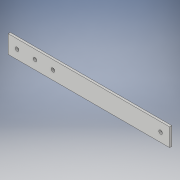
# Autodesk Inventor part: Gearbox Mounting Gusset
Saved by Autodesk Inventor 2018 (Build 220112000, 112)
## iProperties
Created: 2019-01-23
Part Number: Gearbox Mounting Gusset
Material: Generic
Document SubType Name: Modeling
Designer: Gabriel
Density: 1 g/cm^3
Appearance: Default
Author: Gabriel
Autodesk Inventor part; units mm, degrees
ref_plane "YZ Plane" through (0, 0, 0) normal (1, 0, 0) x (0, 1, 0)
ref_plane "XZ Plane" through (0, 0, 0) normal (0, 1, 0) x (-1, 0, 0)
ref_plane "XY Plane" through (0, 0, 0) normal (0, 0, 1) x (1, 0, 0)
sketch "Sketch1" plane through (0, 0, 0) normal (0, 0, 1) x (1, 0, 0)
  line L0 (-12.3524, -19.5597) -> (216.2476, -19.5597)
  line L1 (216.2476, -19.5597) -> (216.2476, -44.9597)
  line L2 (216.2476, -44.9597) -> (-12.3524, -44.9597)
  line L3 (-12.3524, -44.9597) -> (-12.3524, -19.5597)
  point P0 (0, 0)
  dimension "d0" = 228.6
  dimension "d1" = 25.4
  constraints: 8 end point, 2 parallel, 1 horizontal, 1 perpendicular
  measures "d0" distance of L1.end L2.end
  measures "d1" distance of L0.end L1.end
extrude "Extrusion1" add sketch "Sketch1" along normal blind 3.175
sketch "Sketch2" plane through (0, 0, 3.175) normal (0, 0, 1) x (1, 0, 0)
  line L0 (216.2476, -44.9597) -> (216.2476, -19.5597) construction
  line L1 (216.2476, -32.2597) -> (203.5476, -32.2597) construction
  circle A0 centre (203.5476, -32.2597) radius 2.5797
  line L2 (203.5476, -32.2597) -> (51.1476, -32.2597) construction
  circle A1 centre (51.1476, -32.2597) radius 2.5797
  line L3 (51.1476, -32.2597) -> (25.7476, -32.2597) construction
  circle A2 centre (25.7476, -32.2597) radius 2.5797
  line L4 (25.7476, -32.2597) -> (0.3476, -32.2597) construction
  circle A3 centre (0.3476, -32.2597) radius 2.5797
  point P0 (0, 0)
  dimension "d4" = 12.7
  dimension "d5" = 5.1594
  dimension "d6" = 152.4
  dimension "d7" = 5.1594
  dimension "d8" = 25.4
  dimension "d9" = 5.1594
  dimension "d10" = 25.4
  dimension "d11" = 5.1594
  constraints: 8 end point, 4 centre point, 4 coincident, 4 horizontal, 1 midpoint
  measures "d4" distance of L1.start L1.end
  measures "d5" diameter of A0
  measures "d6" distance of L2.start L2.end
  measures "d7" diameter of A1
  measures "d8" distance of L3.start L3.end
  measures "d9" diameter of A2
  measures "d10" distance of L4.start L4.end
  measures "d11" diameter of A3
extrude "Extrusion2" cut sketch "Sketch2" against normal blind 12.7
body "Solid1"
